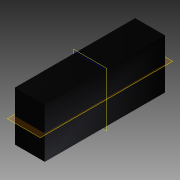
# Autodesk Inventor part: emitter_box
Saved by Autodesk Inventor 2015 SP1 (Build 190203100, 203)
## iProperties
Created: 2015-10-26
Part Number: emitter_box
Material: Generic
Document SubType Name: Modeling
Designer: Alexandre Cherpillod
Density: 1 g/cm^3
Appearance: Fine Textured - Black
Author: Alexandre Cherpillod
Autodesk Inventor part; units mm, degrees
ref_plane "YZ Plane" through (0, 0, 0) normal (1, 0, 0) x (0, 1, 0)
ref_plane "XY Plane" through (0, 0, 0) normal (0, 0, 1) x (1, 0, 0)
sketch "Sketch1" plane through (0, 0, 0) normal (0, 1, 0) x (-1, 0, 0)
  line L0 (0, 0) -> (22.5, 0)
  line L1 (22.5, 0) -> (22.5, -37)
  line L2 (22.5, -37) -> (0, -37)
  line L3 (0, -37) -> (0, 0)
  dimension "d0" = 22.5
  dimension "d1" = 37
  constraints: 8 end point, 2 parallel, 1 horizontal, 1 perpendicular
  measures "d0" distance of L1.end L2.end
  measures "d1" distance of L0.end L1.end
extrude "Extrusion1" add sketch "Sketch1" along normal blind 90.3
ref_plane "Work Plane1" through (0, 45.15, 0) normal (0, 1, 0) x (-1, 0, 0)
ref_plane "Work Plane2" through (-22.5, 0, -18.5) normal (0, 0, 1) x (1, 0, 0)
body "Solid1"
